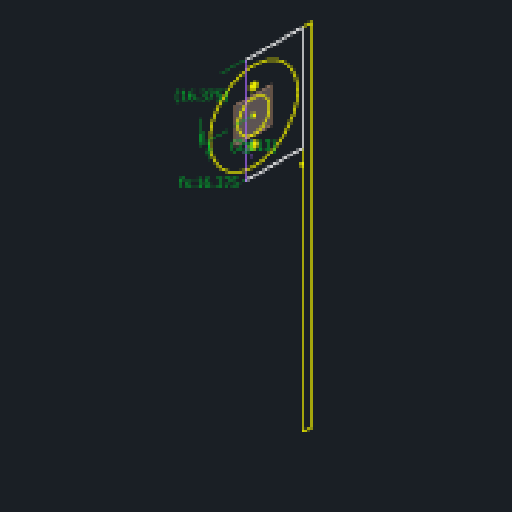
# Autodesk Inventor part: right_motor_mount
Saved by Autodesk Inventor 2023 (Build 270158000, 158)
## iProperties
Created: 2024-04-14
Part Number: right_motor_mount
Material: Generic
Document SubType Name: Modeling
Designer: szymo
Density: 1 g/cm^3
Appearance: Default
Author: szymo
Autodesk Inventor part; units mm, degrees
ref_plane "YZ Plane" through (0, 0, 0) normal (1, 0, 0) x (0, 1, 0)
ref_plane "XZ Plane" through (0, 0, 0) normal (0, 1, 0) x (-1, 0, 0)
ref_plane "XY Plane" through (0, 0, 0) normal (0, 0, 1) x (1, 0, 0)
ref_plane "Work Plane1" through (-24.5, 21.125, 15.375) normal (1, 0, 0) x (0, -1, 0)
sketch "Sketch1" plane through (-24.5, 21.125, 15.375) normal (1, 0, 0) x (0, -1, 0)
  line L0 (-16.375, 15.375) -> (16.375, 15.375)
  line L1 (16.375, 15.375) -> (16.375, -3.0564)
  line L2 (16.375, -3.0564) -> (-16.375, -3.0564)
  line L3 (-16.375, -3.0564) -> (-16.375, 15.375)
  circle A0 centre (0, 0) radius 5 projected
  circle A1 centre (8, 0) radius 1.0564 projected
  circle A2 centre (-8, 0) radius 1.0564 projected
  circle A3 centre (0, 0) radius 5 projected
  circle A4 centre (0, 0) radius 13.7 projected
  line L4 (93.625, 18.375) -> (-16.375, 18.375) projected
  line L5 (-16.375, 18.375) -> (-16.375, 15.375) projected
  line L6 (93.625, 15.375) -> (-16.375, 15.375) projected
  line L7 (93.625, 18.375) -> (93.625, 15.375) projected
  point P0 (21.125, 15.375)
  point P1 (8, -1.0564)
  dimension "d5" = 2.1129
  dimension "d0" = 2
  dimension "d2" = 16.375
  dimension "d3" = 16.375
  dimension "d6" = 1.0564
  constraints: 8 end point, 2 collinear, 2 parallel, 1 horizontal, 1 perpendicular, 1 vertical alignment, 1 other
  measures "d0" distance from line of L2 point (8, -1.056)
  measures "d2" distance from line of L3 A4.centre
  measures "d3" distance from line of L1 A4.centre
  measures "d6" distance of point (8, -1.056) point (8, 0)
extrude "Extrusion1" add sketch "Sketch1" along normal blind 2 and the other way blind 53.2 contours L0 L1 L2 A4 L3 | A4 L2 A0 | A0 L2 | A1 | A2 picked at (7.3146, 4.455) picked at (1.2487, -0.2981)
sketch "Sketch2" plane through (-77.7, 21.125, 15.375) normal (-1, 0, 0) x (0, 0, 1)
  circle A0 centre (0, 0) radius 5 projected
  line L0 (-1.5, 11) -> (1.5, 11) projected
  line L1 (1.5, 11) -> (1.5, 11.5) projected
  line L2 (1.5, 11.5) -> (-1.5, 11.5) projected
  line L3 (-1.5, 11.5) -> (-1.5, 11) projected
  line L4 (1.5, -11.5) -> (-1.5, -11.5) projected
  line L5 (-1.5, -11.5) -> (-1.5, -12) projected
  line L6 (-1.5, -12) -> (1.5, -12) projected
  line L7 (1.5, -12) -> (1.5, -11.5) projected
  line L8 (2, 10.5) -> (-2, 10.5)
  line L9 (-2, 10.5) -> (-2, 12)
  line L10 (-2, 12) -> (2, 12)
  line L11 (2, 12) -> (2, 10.5)
  line L12 (2, -12.5) -> (-2, -12.5)
  line L13 (-2, -12.5) -> (-2, -11)
  line L14 (-2, -11) -> (2, -11)
  line L15 (2, -11) -> (2, -12.5)
  circle A1 centre (0, 0) radius 5.2
  line L16 (3.0564, 16.375) -> (3.0564, -16.375) projected
  line L17 (2, 10.5) -> (3.0564, 10.5)
  line L18 (3.0564, 10.5) -> (3.0564, 12)
  line L19 (3.0564, 12) -> (2, 12)
  line L20 (2, 12) -> (2, 10.5)
  line L21 (2, -12.5) -> (3.0564, -12.5)
  line L22 (3.0564, -12.5) -> (3.0564, -11)
  line L23 (3.0564, -11) -> (2, -11)
  line L24 (2, -11) -> (2, -12.5)
  point P0 (-15.375, -21.125)
  point P1 (2, -11)
  point P2 (3.0564, -12.5)
  point P3 (3.0564, -11)
  point P4 (2, 12)
  point P5 (3.0564, 10.5)
  dimension "d11" = 0.5
  dimension "d12" = 0.5
  dimension "d13" = 0.2
  constraints: 32 end point, 4 parallel, 2 horizontal, 2 perpendicular, 2 point on line, 1 centre point, 6 other
  measures "d11" distance between parallel lines of L0 L8
  measures "d12" distance between parallel lines of L6 L12
  measures "d13" radial gap between concentric circles of A0 A1
ref_plane "Work Plane2" through (-73.7, 7.425, 1.675) normal (-1, 0, 0) x (0, 0, 1)
extrude "Extrusion2" cut sketch "Sketch2" against normal up to surface (4 mm away) contours A0 L16 | A0 L16 A1 | L16 A0 | A0 L16 A1 | L3 L2 L1 L0 | L7 L6 L5 L4 | L8 L9 L10 L11 | L11 L19 L16 L17 | L12 L13 L14 L15 | L15 L23 L16 L21
ref_plane "Work Plane3" through (-73.7, 21.125, 15.375) normal (-1, 0, 0) x (0, 1, 0)
sketch "Sketch3" plane through (-73.7, 21.125, 15.375) normal (-1, 0, 0) x (0, 1, 0)
  line L0 (11, 1.5) -> (11.5, 1.5) projected
  line L1 (11.5, 1.5) -> (11.5, -1.5) projected
  line L2 (11.5, -1.5) -> (11, -1.5) projected
  line L3 (11, -1.5) -> (11, 1.5) projected
  line L4 (-11.5, -1.5) -> (-12, -1.5) projected
  line L5 (-12, -1.5) -> (-12, 1.5) projected
  line L6 (-12, 1.5) -> (-11.5, 1.5) projected
  line L7 (-11.5, 1.5) -> (-11.5, -1.5) projected
  circle A0 centre (0, 0) radius 5 projected
  circle A1 centre (0, 0) radius 13.7 projected
  point P0 (-21.125, 15.375)
ref_plane "Work Plane4" through (-27.2, 7.425, 1.675) normal (1, 0, 0) x (0, 1, 0)
extrude "Extrusion3" cut sketch "Sketch3" against normal up to surface (46.5 mm away) contours L0 L1 L2 L3 | L4 L5 L6 L7 | A0 | A1
ref_plane "Work Plane5" through (-59.9, 21.125, 15.375) normal (-1, 0, 0) x (0, 1, 0)
sketch "Sketch4" plane through (-59.9, 21.125, 15.375) normal (-1, 0, 0) x (0, 1, 0)
  circle A0 centre (0, 0) radius 14.375 projected
  point P0 (-21.125, 15.375)
ref_plane "Work Plane6" through (-32.2, 6.75, 1) normal (1, 0, 0) x (0, 1, 0)
extrude "Extrusion4" cut sketch "Sketch4" against normal up to surface (27.7 mm away)
sketch "Sketch5" plane through (-22.5, 21.125, 15.375) normal (1, 0, 0) x (0, 0, -1)
  circle A0 centre (0, -8) radius 1.0564 projected
  circle A1 centre (0, 8) radius 1.0564 projected
  arc A2 (5.1468, 2.7666) -> (3.0755, 2.3394) centre (5.0543, -2.0206) ccw projected
  arc A3 (3.0755, 2.3394) -> (2.6716, 2.7917) centre (0, 0) ccw projected
  arc A4 (2.6716, 2.7917) -> (3.3299, 4.8016) centre (-1.4371, 5.2501) ccw projected
  arc A5 (3.3299, 4.8016) -> (2.5377, 5.2634) centre (0, 0) ccw projected
  arc A6 (2.5377, 5.2634) -> (1.113, 3.7003) centre (5.2767, 1.3362) ccw projected
  arc A7 (1.113, 3.7003) -> (0.5205, 3.8289) centre (0, 0) ccw projected
  arc A8 (0.5205, 3.8289) -> (-0.1284, 5.8419) centre (-4.2486, 3.4027) ccw projected
  arc A9 (-0.1284, 5.8419) -> (-1.0407, 5.7498) centre (0, 0) ccw projected
  arc A10 (-1.0407, 5.7498) -> (-1.2746, 3.6479) centre (3.4835, 4.1825) ccw projected
  arc A11 (-1.2746, 3.6479) -> (-1.8295, 3.4036) centre (0, 0) ccw projected
  arc A12 (-1.8295, 3.4036) -> (-3.5377, 4.6507) centre (-5.4372, 0.2556) ccw projected
  arc A13 (-3.5377, 4.6507) -> (-4.2216, 4.04) centre (0, 0) ccw projected
  arc A14 (-4.2216, 4.04) -> (-3.1753, 2.202) centre (0.3598, 5.4313) ccw projected
  arc A15 (-3.1753, 2.202) -> (-3.4807, 1.6782) centre (0, 0) ccw projected
  arc A16 (-3.4807, 1.6782) -> (-5.5956, 1.6831) centre (-4.549, -2.9892) ccw projected
  arc A17 (-5.5956, 1.6831) -> (-5.79, 0.787) centre (0, 0) ccw projected
  arc A18 (-5.79, 0.787) -> (-3.8632, -0.0849) centre (-2.9013, 4.6055) ccw projected
  arc A19 (-3.8632, -0.0849) -> (-3.8023, -0.6882) centre (0, 0) ccw projected
  arc A20 (-3.8023, -0.6882) -> (-5.5163, -1.9274) centre (-1.9232, -5.0921) ccw projected
  arc A21 (-5.5163, -1.9274) -> (-5.1468, -2.7666) centre (0, 0) ccw projected
  arc A22 (-5.1468, -2.7666) -> (-3.0755, -2.3394) centre (-5.0543, 2.0206) ccw projected
  arc A23 (-3.0755, -2.3394) -> (-2.6716, -2.7917) centre (0, 0) ccw projected
  arc A24 (-2.6716, -2.7917) -> (-3.3299, -4.8016) centre (1.4371, -5.2501) ccw projected
  arc A25 (-3.3299, -4.8016) -> (-2.5377, -5.2634) centre (0, 0) ccw projected
  arc A26 (-2.5377, -5.2634) -> (-1.113, -3.7003) centre (-5.2767, -1.3362) ccw projected
  arc A27 (-1.113, -3.7003) -> (-0.5205, -3.8289) centre (0, 0) ccw projected
  arc A28 (-0.5205, -3.8289) -> (0.1284, -5.8419) centre (4.2486, -3.4027) ccw projected
  arc A29 (0.1284, -5.8419) -> (1.0407, -5.7498) centre (0, 0) ccw projected
  arc A30 (1.0407, -5.7498) -> (1.2746, -3.6479) centre (-3.4835, -4.1825) ccw projected
  arc A31 (1.2746, -3.6479) -> (1.8295, -3.4036) centre (0, 0) ccw projected
  arc A32 (1.8295, -3.4036) -> (3.5377, -4.6507) centre (5.4372, -0.2556) ccw projected
  arc A33 (3.5377, -4.6507) -> (4.2216, -4.04) centre (0, 0) ccw projected
  arc A34 (4.2216, -4.04) -> (3.1753, -2.202) centre (-0.3598, -5.4313) ccw projected
  arc A35 (3.1753, -2.202) -> (3.4807, -1.6782) centre (0, 0) ccw projected
  arc A36 (3.4807, -1.6782) -> (5.5956, -1.6831) centre (4.549, 2.9892) ccw projected
  arc A37 (5.5956, -1.6831) -> (5.79, -0.787) centre (0, 0) ccw projected
  arc A38 (5.79, -0.787) -> (3.8632, 0.0849) centre (2.9013, -4.6055) ccw projected
  arc A39 (3.8632, 0.0849) -> (3.8023, 0.6882) centre (0, 0) ccw projected
  arc A40 (3.8023, 0.6882) -> (5.5163, 1.9274) centre (1.9232, 5.0921) ccw projected
  arc A41 (5.5163, 1.9274) -> (5.1468, 2.7666) centre (0, 0) ccw projected
  circle A42 centre (0, 0) radius 5.8433
  circle A43 centre (0, 0) radius 6.3433
  point P0 (15.375, -21.125)
  dimension "d20" = 0.5
  constraints: 2 centre point, 1 coincident
  measures "d20" radial gap between concentric circles of A42 A43
extrude "Extrusion5" cut sketch "Sketch5" along normal mid plane 10 contours A0 | A1 | A41 A40 A39 A38 A37 A36 A35 A34 A33 A32 A31 A30 A29 A28 A27 A26 A25 A24 A23 A22 A21 A20 A19 A18 A17 A16 A15 A14 A13 A12 A11 A10 A9 A8 A7 A6 A5 A4 A3 A2 | A2 A3 A4 A42 | A42 A38 A39 A40 | A6 A7 A8 A42 | A42 A34 A35 A36 | A10 A11 A12 A42 | A42 A30 A31 A32 | A14 A15 A16 A42 | A42 A26 A27 A28 | A18 A19 A20 A42 | A42 A22 A23 A24 | A43
equation "\"d3\" = d2"
equation "\"d6\" = 0.5 * d5"
body "Solid1"
